Autodesk Inventor part; units mm, degrees
(part 2 of 3)
sketch "Sketch4" plane through (360.9, 0, 0) normal (0, 0, 1) x (1, 0, 0)
  line L0 (43.995, -13.335) -> (40.185, -13.335) projected
  line L1 (40.185, -13.335) -> (40.185, -1.905) projected
  line L2 (40.185, -1.905) -> (43.995, -1.905) projected
  line L3 (43.995, -1.905) -> (43.995, -13.335) projected
  circle A0 centre (38.28, -15.24) radius 1.078 projected
  circle A1 centre (45.9, 0) radius 1.078 projected
  circle A2 centre (45.9, -15.24) radius 1.078 projected
  circle A3 centre (38.28, 0) radius 1.078 projected
  line L4 (55.005, -48.5) -> (57.005, -48.5) projected
  line L5 (57.005, -48.5) -> (57.005, -45) projected
  line L6 (57.005, -45) -> (60.18, -45) projected
  line L7 (60.18, -45) -> (60.18, -35) projected
  line L8 (60.18, -35) -> (57.005, -35) projected
  line L9 (57.005, -35) -> (57.005, -25) projected
  line L10 (57.005, -25) -> (60.18, -25) projected
  line L11 (60.18, -25) -> (60.18, -15) projected
  line L12 (60.18, -15) -> (57.005, -15) projected
  line L13 (57.005, -15) -> (57.005, -5) projected
  line L14 (57.005, -5) -> (60.18, -5) projected
  line L15 (60.18, -5) -> (60.18, 5) projected
  line L16 (60.18, 5) -> (57.005, 5) projected
  line L17 (57.005, 5) -> (57.005, 15) projected
  line L18 (57.005, 15) -> (60.18, 15) projected
  line L19 (60.18, 15) -> (60.18, 25) projected
  line L20 (60.18, 25) -> (57.005, 25) projected
  line L21 (57.005, 25) -> (57.005, 35) projected
  line L22 (57.005, 35) -> (60.18, 35) projected
  line L23 (60.18, 35) -> (60.18, 45) projected
  line L24 (60.18, 45) -> (57.005, 45) projected
  line L25 (57.005, 45) -> (57.005, 48.5) projected
  line L26 (57.005, 48.5) -> (55.005, 48.5) projected
  line L27 (55.005, 48.5) -> (55.005, 47.25) projected
  line L28 (55.005, 47.25) -> (52.505, 47.25) projected
  line L29 (52.505, 47.25) -> (52.505, 48.5) projected
  line L30 (52.505, 48.5) -> (46.18, 48.5) projected
  line L31 (46.18, 48.5) -> (46.18, 51.5) projected
  line L32 (46.18, 51.5) -> (52.505, 51.5) projected
  line L33 (52.505, 51.5) -> (52.505, 52.75) projected
  line L34 (52.505, 52.75) -> (55.005, 52.75) projected
  line L35 (55.005, 52.75) -> (55.005, 51.5) projected
  line L36 (55.005, 51.5) -> (57.005, 51.5) projected
  line L37 (57.005, 51.5) -> (57.005, 55) projected
  line L38 (57.005, 55) -> (60.18, 55) projected
  line L39 (60.18, 55) -> (60.18, 65) projected
  line L40 (60.18, 65) -> (57.005, 65) projected
  line L41 (57.005, 65) -> (57.005, 75) projected
  line L42 (57.005, 75) -> (60.18, 75) projected
  line L43 (60.18, 75) -> (60.18, 86.825) projected
  line L44 (55.18, 86.825) -> (60.18, 86.825) projected
  line L45 (55.18, 90) -> (55.18, 86.825) projected
  line L46 (45.18, 90) -> (55.18, 90) projected
  line L47 (45.18, 86.825) -> (45.18, 90) projected
  line L48 (45.18, 86.825) -> (35.18, 86.825) projected
  line L49 (35.18, 90) -> (35.18, 86.825) projected
  line L50 (25.18, 90) -> (35.18, 90) projected
  line L51 (25.18, 86.825) -> (25.18, 90) projected
  line L52 (25.18, 86.825) -> (15.18, 86.825) projected
  line L53 (15.18, 90) -> (15.18, 86.825) projected
  line L54 (5.18, 90) -> (15.18, 90) projected
  line L55 (5.18, 86.825) -> (5.18, 90) projected
  line L56 (5.18, 86.825) -> (-4.82, 86.825) projected
  line L57 (-4.82, 90) -> (-4.82, 86.825) projected
  line L58 (-14.82, 90) -> (-4.82, 90) projected
  line L59 (-14.82, 86.825) -> (-14.82, 90) projected
  line L60 (-14.82, 86.825) -> (-24.82, 86.825) projected
  line L61 (-24.82, 90) -> (-24.82, 86.825) projected
  line L62 (-34.82, 90) -> (-24.82, 90) projected
  line L63 (-34.82, 86.825) -> (-34.82, 90) projected
  line L64 (-34.82, 86.825) -> (-44.82, 86.825) projected
  line L65 (-44.82, 90) -> (-44.82, 86.825) projected
  line L66 (-54.82, 90) -> (-44.82, 90) projected
  line L67 (-54.82, 86.825) -> (-54.82, 90) projected
  line L68 (-54.82, 86.825) -> (-59.82, 86.825) projected
  line L69 (-59.82, 75) -> (-59.82, 86.825) projected
  line L70 (-56.645, 75) -> (-59.82, 75) projected
  line L71 (-56.645, 75) -> (-56.645, 65) projected
  line L72 (-59.82, 65) -> (-56.645, 65) projected
  line L73 (-59.82, 55) -> (-59.82, 65) projected
  line L74 (-56.645, 55) -> (-59.82, 55) projected
  line L75 (-56.645, 55) -> (-56.645, 45) projected
  line L76 (-59.82, 45) -> (-56.645, 45) projected
  line L77 (-59.82, 35) -> (-59.82, 45) projected
  line L78 (-56.645, 35) -> (-59.82, 35) projected
  line L79 (-56.645, 35) -> (-56.645, 25) projected
  line L80 (-59.82, 25) -> (-56.645, 25) projected
  line L81 (-59.82, 15) -> (-59.82, 25) projected
  line L82 (-56.645, 15) -> (-59.82, 15) projected
  line L83 (-56.645, 15) -> (-56.645, 5) projected
  line L84 (-59.82, 5) -> (-56.645, 5) projected
  line L85 (-59.82, -5) -> (-59.82, 5) projected
  line L86 (-56.645, -5) -> (-59.82, -5) projected
  line L87 (-56.645, -5) -> (-56.645, -15) projected
  line L88 (-59.82, -15) -> (-56.645, -15) projected
  line L89 (-59.82, -25) -> (-59.82, -15) projected
  line L90 (-56.645, -25) -> (-59.82, -25) projected
  line L91 (-56.645, -25) -> (-56.645, -35) projected
  line L92 (-59.82, -35) -> (-56.645, -35) projected
  line L93 (-59.82, -45) -> (-59.82, -35) projected
  line L94 (-56.645, -45) -> (-59.82, -45) projected
  line L95 (-56.645, -45) -> (-56.645, -55) projected
  line L96 (-59.82, -55) -> (-56.645, -55) projected
  line L97 (-59.82, -65) -> (-59.82, -55) projected
  line L98 (-56.645, -65) -> (-59.82, -65) projected
  line L99 (-56.645, -65) -> (-56.645, -75) projected
  line L100 (-59.82, -75) -> (-56.645, -75) projected
  line L101 (-59.82, -75) -> (-59.82, -86.825) projected
  line L102 (-59.82, -86.825) -> (-54.82, -86.825) projected
  line L103 (-54.82, -86.825) -> (-54.82, -90) projected
  line L104 (-54.82, -90) -> (-44.82, -90) projected
  line L105 (-44.82, -90) -> (-44.82, -86.825) projected
  line L106 (-44.82, -86.825) -> (-34.82, -86.825) projected
  line L107 (-34.82, -86.825) -> (-34.82, -90) projected
  line L108 (-34.82, -90) -> (-24.82, -90) projected
  line L109 (-24.82, -90) -> (-24.82, -86.825) projected
  line L110 (-24.82, -86.825) -> (-14.82, -86.825) projected
  line L111 (-14.82, -86.825) -> (-14.82, -90) projected
  line L112 (-14.82, -90) -> (-4.82, -90) projected
  line L113 (-4.82, -90) -> (-4.82, -86.825) projected
  line L114 (-4.82, -86.825) -> (5.18, -86.825) projected
  line L115 (5.18, -86.825) -> (5.18, -90) projected
  line L116 (5.18, -90) -> (15.18, -90) projected
  line L117 (15.18, -90) -> (15.18, -86.825) projected
  line L118 (15.18, -86.825) -> (25.18, -86.825) projected
  line L119 (25.18, -86.825) -> (25.18, -90) projected
  line L120 (25.18, -90) -> (35.18, -90) projected
  line L121 (35.18, -90) -> (35.18, -86.825) projected
  line L122 (35.18, -86.825) -> (45.18, -86.825) projected
  line L123 (45.18, -86.825) -> (45.18, -90) projected
  line L124 (45.18, -90) -> (55.18, -90) projected
  line L125 (55.18, -90) -> (55.18, -86.825) projected
  line L126 (55.18, -86.825) -> (60.18, -86.825) projected
  line L127 (60.18, -86.825) -> (60.18, -75) projected
  line L128 (60.18, -75) -> (57.005, -75) projected
  line L129 (57.005, -75) -> (57.005, -65) projected
  line L130 (57.005, -65) -> (60.18, -65) projected
  line L131 (60.18, -65) -> (60.18, -55) projected
  line L132 (60.18, -55) -> (57.005, -55) projected
  line L133 (57.005, -55) -> (57.005, -51.5) projected
  line L134 (57.005, -51.5) -> (55.005, -51.5) projected
  line L135 (55.005, -51.5) -> (55.005, -52.75) projected
  line L136 (55.005, -52.75) -> (52.505, -52.75) projected
  line L137 (52.505, -52.75) -> (52.505, -51.5) projected
  line L138 (52.505, -51.5) -> (46.18, -51.5) projected
  line L139 (46.18, -51.5) -> (46.18, -48.5) projected
  line L140 (46.18, -48.5) -> (52.505, -48.5) projected
  line L141 (52.505, -48.5) -> (52.505, -47.25) projected
  line L142 (52.505, -47.25) -> (55.005, -47.25) projected
  line L143 (55.005, -47.25) -> (55.005, -48.5) projected
  circle A4 centre (23.1772, -27.4451) radius 3 projected
  circle A5 centre (-22.8172, 54) radius 3 projected
  circle A6 centre (23.1772, 27.4451) radius 3 projected
  circle A7 centre (-22.8172, -54) radius 3 projected
  circle A8 centre (-14.82, 8.175) radius 11 projected
  line L144 (45.06, 90.12) -> (55.3, 90.12)
  line L145 (55.3, 90.12) -> (55.3, 86.945)
  line L146 (55.3, 86.945) -> (60.3, 86.945)
  line L147 (60.3, 86.945) -> (60.3, 74.88)
  line L148 (60.3, 74.88) -> (57.125, 74.88)
  line L149 (57.125, 74.88) -> (57.125, 65.12)
  line L150 (57.125, 65.12) -> (60.3, 65.12)
  line L151 (60.3, 65.12) -> (60.3, 54.88)
  line L152 (60.3, 54.88) -> (57.125, 54.88)
  line L153 (57.125, 54.88) -> (57.125, 51.38)
  line L154 (57.125, 51.38) -> (54.885, 51.38)
  line L155 (54.885, 51.38) -> (54.885, 52.63)
  line L156 (54.885, 52.63) -> (52.625, 52.63)
  line L157 (52.625, 52.63) -> (52.625, 51.38)
  line L158 (52.625, 51.38) -> (46.3, 51.38)
  line L159 (46.3, 51.38) -> (46.3, 48.62)
  line L160 (46.3, 48.62) -> (52.625, 48.62)
  line L161 (52.625, 48.62) -> (52.625, 47.37)
  line L162 (52.625, 47.37) -> (54.885, 47.37)
  line L163 (54.885, 47.37) -> (54.885, 48.62)
  line L164 (54.885, 48.62) -> (57.125, 48.62)
  line L165 (57.125, 48.62) -> (57.125, 45.12)
  line L166 (57.125, 45.12) -> (60.3, 45.12)
  line L167 (60.3, 45.12) -> (60.3, 34.88)
  line L168 (60.3, 34.88) -> (57.125, 34.88)
  line L169 (57.125, 34.88) -> (57.125, 25.12)
  line L170 (57.125, 25.12) -> (60.3, 25.12)
  line L171 (60.3, 25.12) -> (60.3, 14.88)
  line L172 (60.3, 14.88) -> (57.125, 14.88)
  line L173 (57.125, 14.88) -> (57.125, 5.12)
  line L174 (57.125, 5.12) -> (60.3, 5.12)
  line L175 (60.3, 5.12) -> (60.3, -5.12)
  line L176 (60.3, -5.12) -> (57.125, -5.12)
  line L177 (57.125, -5.12) -> (57.125, -14.88)
  line L178 (57.125, -14.88) -> (60.3, -14.88)
  line L179 (60.3, -14.88) -> (60.3, -25.12)
  line L180 (60.3, -25.12) -> (57.125, -25.12)
  line L181 (57.125, -25.12) -> (57.125, -34.88)
  line L182 (57.125, -34.88) -> (60.3, -34.88)
  line L183 (60.3, -34.88) -> (60.3, -45.12)
  line L184 (60.3, -45.12) -> (57.125, -45.12)
  line L185 (57.125, -45.12) -> (57.125, -48.62)
  line L186 (57.125, -48.62) -> (54.885, -48.62)
  line L187 (54.885, -48.62) -> (54.885, -47.37)
  line L188 (54.885, -47.37) -> (52.625, -47.37)
  line L189 (52.625, -47.37) -> (52.625, -48.62)
  line L190 (52.625, -48.62) -> (46.3, -48.62)
  line L191 (46.3, -48.62) -> (46.3, -51.38)
  line L192 (46.3, -51.38) -> (52.625, -51.38)
  line L193 (52.625, -51.38) -> (52.625, -52.63)
  line L194 (52.625, -52.63) -> (54.885, -52.63)
  line L195 (54.885, -52.63) -> (54.885, -51.38)
  line L196 (54.885, -51.38) -> (57.125, -51.38)
  line L197 (57.125, -51.38) -> (57.125, -54.88)
  line L198 (57.125, -54.88) -> (60.3, -54.88)
  line L199 (60.3, -54.88) -> (60.3, -65.12)
  line L200 (60.3, -65.12) -> (57.125, -65.12)
  line L201 (57.125, -65.12) -> (57.125, -74.88)
  line L202 (57.125, -74.88) -> (60.3, -74.88)
  line L203 (60.3, -74.88) -> (60.3, -86.945)
  line L204 (60.3, -86.945) -> (55.3, -86.945)
  line L205 (55.3, -86.945) -> (55.3, -90.12)
  line L206 (55.3, -90.12) -> (45.06, -90.12)
  line L207 (45.06, -90.12) -> (45.06, -86.945)
  line L208 (45.06, -86.945) -> (35.3, -86.945)
  line L209 (35.3, -86.945) -> (35.3, -90.12)
  line L210 (35.3, -90.12) -> (25.06, -90.12)
  line L211 (25.06, -90.12) -> (25.06, -86.945)
  line L212 (25.06, -86.945) -> (15.3, -86.945)
  line L213 (15.3, -86.945) -> (15.3, -90.12)
  line L214 (15.3, -90.12) -> (5.06, -90.12)
  line L215 (5.06, -90.12) -> (5.06, -86.945)
  line L216 (5.06, -86.945) -> (-4.7, -86.945)
  line L217 (-4.7, -86.945) -> (-4.7, -90.12)
  line L218 (-4.7, -90.12) -> (-14.94, -90.12)
  line L219 (-14.94, -90.12) -> (-14.94, -86.945)
  line L220 (-14.94, -86.945) -> (-24.7, -86.945)
  line L221 (-24.7, -86.945) -> (-24.7, -90.12)
  line L222 (-24.7, -90.12) -> (-34.94, -90.12)
  line L223 (-34.94, -90.12) -> (-34.94, -86.945)
  line L224 (-34.94, -86.945) -> (-44.7, -86.945)
  line L225 (-44.7, -86.945) -> (-44.7, -90.12)
  line L226 (-44.7, -90.12) -> (-54.94, -90.12)
  line L227 (-54.94, -90.12) -> (-54.94, -86.945)
  line L228 (-54.94, -86.945) -> (-59.94, -86.945)
  line L229 (-59.94, -86.945) -> (-59.94, -74.88)
  line L230 (-59.94, -74.88) -> (-56.765, -74.88)
  line L231 (-56.765, -74.88) -> (-56.765, -65.12)
  line L232 (-56.765, -65.12) -> (-59.94, -65.12)
  line L233 (-59.94, -65.12) -> (-59.94, -54.88)
  line L234 (-59.94, -54.88) -> (-56.765, -54.88)
  line L235 (-56.765, -54.88) -> (-56.765, -45.12)
  line L236 (-56.765, -45.12) -> (-59.94, -45.12)
  line L237 (-59.94, -45.12) -> (-59.94, -34.88)
  line L238 (-59.94, -34.88) -> (-56.765, -34.88)
  line L239 (-56.765, -34.88) -> (-56.765, -25.12)
  line L240 (-56.765, -25.12) -> (-59.94, -25.12)
  line L241 (-59.94, -25.12) -> (-59.94, -14.88)
  line L242 (-59.94, -14.88) -> (-56.765, -14.88)
  line L243 (-56.765, -14.88) -> (-56.765, -5.12)
  line L244 (-56.765, -5.12) -> (-59.94, -5.12)
  line L245 (-59.94, -5.12) -> (-59.94, 5.12)
  line L246 (-59.94, 5.12) -> (-56.765, 5.12)
  line L247 (-56.765, 5.12) -> (-56.765, 14.88)
  line L248 (-56.765, 14.88) -> (-59.94, 14.88)
  line L249 (-59.94, 14.88) -> (-59.94, 25.12)
  line L250 (-59.94, 25.12) -> (-56.765, 25.12)
  line L251 (-56.765, 25.12) -> (-56.765, 34.88)
  line L252 (-56.765, 34.88) -> (-59.94, 34.88)
  line L253 (-59.94, 34.88) -> (-59.94, 45.12)
  line L254 (-59.94, 45.12) -> (-56.765, 45.12)
  line L255 (-56.765, 45.12) -> (-56.765, 54.88)
  line L256 (-56.765, 54.88) -> (-59.94, 54.88)
  line L257 (-59.94, 54.88) -> (-59.94, 65.12)
  line L258 (-59.94, 65.12) -> (-56.765, 65.12)
  line L259 (-56.765, 65.12) -> (-56.765, 74.88)
  line L260 (-56.765, 74.88) -> (-59.94, 74.88)
  line L261 (-59.94, 74.88) -> (-59.94, 86.945)
  line L262 (-59.94, 86.945) -> (-54.94, 86.945)
  line L263 (-54.94, 86.945) -> (-54.94, 90.12)
  line L264 (-54.94, 90.12) -> (-44.7, 90.12)
  line L265 (-44.7, 90.12) -> (-44.7, 86.945)
  line L266 (-44.7, 86.945) -> (-34.94, 86.945)
  line L267 (-34.94, 86.945) -> (-34.94, 90.12)
  line L268 (-34.94, 90.12) -> (-24.7, 90.12)
  line L269 (-24.7, 90.12) -> (-24.7, 86.945)
  line L270 (-24.7, 86.945) -> (-14.94, 86.945)
  line L271 (-14.94, 86.945) -> (-14.94, 90.12)
  line L272 (-14.94, 90.12) -> (-4.7, 90.12)
  line L273 (-4.7, 90.12) -> (-4.7, 86.945)
  line L274 (-4.7, 86.945) -> (5.06, 86.945)
  line L275 (5.06, 86.945) -> (5.06, 90.12)
  line L276 (5.06, 90.12) -> (15.3, 90.12)
  line L277 (15.3, 90.12) -> (15.3, 86.945)
  line L278 (15.3, 86.945) -> (25.06, 86.945)
  line L279 (25.06, 86.945) -> (25.06, 90.12)
  line L280 (25.06, 90.12) -> (35.3, 90.12)
  line L281 (35.3, 90.12) -> (35.3, 86.945)
  line L282 (35.3, 86.945) -> (45.06, 86.945)
  line L283 (45.06, 86.945) -> (45.06, 90.12)
  circle A9 centre (45.9, 0) radius 0.958
  circle A10 centre (38.28, 0) radius 1.198
  line L284 (43.875, -13.215) -> (40.305, -13.215)
  line L285 (40.305, -13.215) -> (40.305, -2.025)
  line L286 (40.305, -2.025) -> (43.875, -2.025)
  line L287 (43.875, -2.025) -> (43.875, -13.215)
  circle A11 centre (45.9, -15.24) radius 0.958
  circle A12 centre (38.28, -15.24) radius 0.958
  circle A13 centre (23.1772, -27.4451) radius 2.88
  circle A14 centre (23.1772, 27.4451) radius 2.88
  circle A15 centre (-14.82, 8.175) radius 10.88
  circle A16 centre (-22.8172, -54) radius 2.88
  circle A17 centre (-22.8172, 54) radius 2.88
  point P0 (-360.9, 0)
  dimension "d28" = 0.12
  dimension "d29" = 0.12
  dimension "d30" = 0.12
  dimension "d31" = 0.12
  dimension "d32" = 0.12
  dimension "d33" = 0.12
  dimension "d34" = 0.12
  dimension "d35" = 0.12
  dimension "d36" = 0.12
  dimension "d37" = 0.12
  dimension "d38" = 0.12
  constraints: 288 end point, 9 centre point, 142 other
  measures "d28" distance between parallel lines of L47 L283
  measures "d29" radial gap between concentric circles of A1 A9
  measures "d30" radial gap between concentric circles of A3 A10
  measures "d31" distance between parallel lines of L3 L287
  measures "d32" radial gap between concentric circles of A2 A11
  measures "d33" radial gap between concentric circles of A0 A12
  measures "d34" radial gap between concentric circles of A4 A13
  measures "d35" radial gap between concentric circles of A6 A14
  measures "d36" radial gap between concentric circles of A8 A15
  measures "d37" radial gap between concentric circles of A7 A16
  measures "d38" radial gap between concentric circles of A5 A17
extrude "Extrusion4" add sketch "Sketch4" along normal blind 3.175 contours L0 L1 L2 L3 | A0 | A1 | A2 | L143 L142 L141 L140 L139 L138 L137 L136 L135 L134 L133 L132 L131 L130 L129 L128 L127 L126 L125 L124 L123 L122 L121 L120 L119 L118 L117 L116 L115 L114 L113 L112 L111 L110 L109 L108 L107 L106 L105 L104 L103 L102 L101 L100 L99 L98 L97 L96 L95 L94 L93 L92 L91 L90 L89 L88 L87 L86 L85 L84 L83 L82 L81 L80 L79 L78 L77 L76 L75 L74 L73 L72 L71 L70 L69 L68 L67 L66 L65 L64 L63 L62 L61 L60 L59 L58 L57 L56 L55 L54 L53 L52 L51 L50 L49 L48 L47 L46 L45 L44 L43 L42 L41 L40 L39 L38 L37 L36 L35 L34 L33 L32 L31 L30 L29 L28 L27 L26 L25 L24 L23 L22 L21 L20 L19 L18 L17 L16 L15 L14 L13 L12 L11 L10 L9 L8 L7 L6 L5 L4 | A4 | A5 | A6 | A7 | A8 | A10
ref_plane "Work Plane4" through (120.3, -150.3, 0) normal (0, 0, 1) x (0, -1, 0)
sketch "Sketch5" plane through (120.3, -150.3, 0) normal (0, 0, 1) x (0, -1, 0)
  line L0 (56.885, 55.06) -> (60.06, 55.06) projected
  line L1 (60.06, 55.06) -> (60.06, 60.06) projected
  line L2 (60.06, 60.06) -> (55.06, 60.06) projected
  line L3 (55.06, 60.06) -> (55.06, 56.885) projected
  line L4 (55.06, 56.885) -> (45.06, 56.885) projected
  line L5 (45.06, 56.885) -> (45.06, 60.06) projected
  line L6 (45.06, 60.06) -> (35.06, 60.06) projected
  line L7 (35.06, 60.06) -> (35.06, 56.885) projected
  line L8 (35.06, 56.885) -> (25.06, 56.885) projected
  line L9 (25.06, 56.885) -> (25.06, 60.06) projected
  line L10 (25.06, 60.06) -> (15.06, 60.06) projected
  line L11 (15.06, 60.06) -> (15.06, 56.885) projected
  line L12 (15.06, 56.885) -> (5.06, 56.885) projected
  line L13 (5.06, 56.885) -> (5.06, 60.06) projected
  line L14 (5.06, 60.06) -> (-4.94, 60.06) projected
  line L15 (-4.94, 60.06) -> (-4.94, 56.885) projected
  line L16 (-4.94, 56.885) -> (-14.94, 56.885) projected
  line L17 (-14.94, 56.885) -> (-14.94, 60.06) projected
  line L18 (-14.94, 60.06) -> (-24.94, 60.06) projected
  line L19 (-24.94, 60.06) -> (-24.94, 56.885) projected
  line L20 (-24.94, 56.885) -> (-34.94, 56.885) projected
  line L21 (-34.94, 56.885) -> (-34.94, 60.06) projected
  line L22 (-34.94, 60.06) -> (-44.94, 60.06) projected
  line L23 (-44.94, 60.06) -> (-44.94, 56.885) projected
  line L24 (-44.94, 56.885) -> (-54.94, 56.885) projected
  line L25 (-54.94, 56.885) -> (-54.94, 60.06) projected
  line L26 (-54.94, 60.06) -> (-59.94, 60.06) projected
  line L27 (-59.94, 60.06) -> (-59.94, 55.06) projected
  line L28 (-59.94, 55.06) -> (-56.765, 55.06) projected
  line L29 (-56.765, 55.06) -> (-56.765, 45.06) projected
  line L30 (-56.765, 45.06) -> (-59.94, 45.06) projected
  line L31 (-59.94, 45.06) -> (-59.94, 35.06) projected
  line L32 (-59.94, 35.06) -> (-56.765, 35.06) projected
  line L33 (-56.765, 35.06) -> (-56.765, 25.06) projected
  line L34 (-56.765, 25.06) -> (-59.94, 25.06) projected
  line L35 (-59.94, 25.06) -> (-59.94, 15.06) projected
  line L36 (-59.94, 15.06) -> (-56.765, 15.06) projected
  line L37 (-56.765, 15.06) -> (-56.765, 5.06) projected
  line L38 (-56.765, 5.06) -> (-59.94, 5.06) projected
  line L39 (-59.94, 5.06) -> (-59.94, -4.94) projected
  line L40 (-59.94, -4.94) -> (-56.765, -4.94) projected
  line L41 (-56.765, -4.94) -> (-56.765, -14.94) projected
  line L42 (-56.765, -14.94) -> (-59.94, -14.94) projected
  line L43 (-59.94, -14.94) -> (-59.94, -24.94) projected
  line L44 (-59.94, -24.94) -> (-56.765, -24.94) projected
  line L45 (-56.765, -24.94) -> (-56.765, -34.94) projected
  line L46 (-56.765, -34.94) -> (-59.94, -34.94) projected
  line L47 (-59.94, -34.94) -> (-59.94, -44.94) projected
  line L48 (-59.94, -44.94) -> (-56.765, -44.94) projected
  line L49 (-56.765, -44.94) -> (-56.765, -54.94) projected
  line L50 (-56.765, -54.94) -> (-59.94, -54.94) projected
  line L51 (-59.94, -54.94) -> (-59.94, -59.94) projected
  line L52 (-59.94, -59.94) -> (-54.94, -59.94) projected
  line L53 (-54.94, -59.94) -> (-54.94, -56.765) projected
  line L54 (-54.94, -56.765) -> (-44.94, -56.765) projected
  line L55 (-44.94, -56.765) -> (-44.94, -59.94) projected
  line L56 (-44.94, -59.94) -> (-34.94, -59.94) projected
  line L57 (-34.94, -59.94) -> (-34.94, -56.765) projected
  line L58 (-34.94, -56.765) -> (-24.94, -56.765) projected
  line L59 (-24.94, -56.765) -> (-24.94, -59.94) projected
  line L60 (-24.94, -59.94) -> (-14.94, -59.94) projected
  line L61 (-14.94, -59.94) -> (-14.94, -56.765) projected
  line L62 (-14.94, -56.765) -> (-4.94, -56.765) projected
  line L63 (-4.94, -56.765) -> (-4.94, -59.94) projected
  line L64 (-4.94, -59.94) -> (5.06, -59.94) projected
  line L65 (5.06, -59.94) -> (5.06, -56.765) projected
  line L66 (5.06, -56.765) -> (15.06, -56.765) projected
  line L67 (15.06, -56.765) -> (15.06, -59.94) projected
  line L68 (15.06, -59.94) -> (25.06, -59.94) projected
  line L69 (25.06, -59.94) -> (25.06, -56.765) projected
  line L70 (25.06, -56.765) -> (35.06, -56.765) projected
  line L71 (35.06, -56.765) -> (35.06, -59.94) projected
  line L72 (35.06, -59.94) -> (45.06, -59.94) projected
  line L73 (45.06, -59.94) -> (45.06, -56.765) projected
  line L74 (45.06, -56.765) -> (55.06, -56.765) projected
  line L75 (55.06, -56.765) -> (55.06, -59.94) projected
  line L76 (55.06, -59.94) -> (60.06, -59.94) projected
  line L77 (60.06, -59.94) -> (60.06, -54.94) projected
  line L78 (60.06, -54.94) -> (56.885, -54.94) projected
  line L79 (56.885, -54.94) -> (56.885, -44.94) projected
  line L80 (56.885, -44.94) -> (60.06, -44.94) projected
  line L81 (60.06, -44.94) -> (60.06, -34.94) projected
  line L82 (60.06, -34.94) -> (56.885, -34.94) projected
  line L83 (56.885, -34.94) -> (56.885, -24.94) projected
  line L84 (56.885, -24.94) -> (60.06, -24.94) projected
  line L85 (60.06, -24.94) -> (60.06, -14.94) projected
  line L86 (60.06, -14.94) -> (56.885, -14.94) projected
  line L87 (56.885, -14.94) -> (56.885, -4.94) projected
  line L88 (56.885, -4.94) -> (60.06, -4.94) projected
  line L89 (60.06, -4.94) -> (60.06, 5.06) projected
  line L90 (60.06, 5.06) -> (56.885, 5.06) projected
  line L91 (56.885, 5.06) -> (56.885, 15.06) projected
  line L92 (56.885, 15.06) -> (60.06, 15.06) projected
  line L93 (60.06, 15.06) -> (60.06, 25.06) projected
  line L94 (60.06, 25.06) -> (56.885, 25.06) projected
  line L95 (56.885, 25.06) -> (56.885, 35.06) projected
  line L96 (56.885, 35.06) -> (60.06, 35.06) projected
  line L97 (60.06, 35.06) -> (60.06, 45.06) projected
  line L98 (60.06, 45.06) -> (56.885, 45.06) projected
  line L99 (56.885, 45.06) -> (56.885, 55.06) projected
  line L100 (57.005, -45.06) -> (57.005, -54.82)
  line L101 (57.005, -54.82) -> (60.18, -54.82)
  line L102 (60.18, -54.82) -> (60.18, -60.06)
  line L103 (60.18, -60.06) -> (54.94, -60.06)
  line L104 (54.94, -60.06) -> (54.94, -56.885)
  line L105 (54.94, -56.885) -> (45.18, -56.885)
  line L106 (45.18, -56.885) -> (45.18, -60.06)
  line L107 (45.18, -60.06) -> (34.94, -60.06)
  line L108 (34.94, -60.06) -> (34.94, -56.885)
  line L109 (34.94, -56.885) -> (25.18, -56.885)
  line L110 (25.18, -56.885) -> (25.18, -60.06)
  line L111 (25.18, -60.06) -> (14.94, -60.06)
  line L112 (14.94, -60.06) -> (14.94, -56.885)
  line L113 (14.94, -56.885) -> (5.18, -56.885)
  line L114 (5.18, -56.885) -> (5.18, -60.06)
  line L115 (5.18, -60.06) -> (-5.06, -60.06)
  line L116 (-5.06, -60.06) -> (-5.06, -56.885)
  line L117 (-5.06, -56.885) -> (-14.82, -56.885)
  line L118 (-14.82, -56.885) -> (-14.82, -60.06)
  line L119 (-14.82, -60.06) -> (-25.06, -60.06)
  line L120 (-25.06, -60.06) -> (-25.06, -56.885)
  line L121 (-25.06, -56.885) -> (-34.82, -56.885)
  line L122 (-34.82, -56.885) -> (-34.82, -60.06)
  line L123 (-34.82, -60.06) -> (-45.06, -60.06)
  line L124 (-45.06, -60.06) -> (-45.06, -56.885)
  line L125 (-45.06, -56.885) -> (-54.82, -56.885)
  line L126 (-54.82, -56.885) -> (-54.82, -60.06)
  line L127 (-54.82, -60.06) -> (-60.06, -60.06)
  line L128 (-60.06, -60.06) -> (-60.06, -54.82)
  line L129 (-60.06, -54.82) -> (-56.885, -54.82)
  line L130 (-56.885, -54.82) -> (-56.885, -45.06)
  line L131 (-56.885, -45.06) -> (-60.06, -45.06)
  line L132 (-60.06, -45.06) -> (-60.06, -34.82)
  line L133 (-60.06, -34.82) -> (-56.885, -34.82)
  line L134 (-56.885, -34.82) -> (-56.885, -25.06)
  line L135 (-56.885, -25.06) -> (-60.06, -25.06)
  line L136 (-60.06, -25.06) -> (-60.06, -14.82)
  line L137 (-60.06, -14.82) -> (-56.885, -14.82)
  line L138 (-56.885, -14.82) -> (-56.885, -5.06)
  line L139 (-56.885, -5.06) -> (-60.06, -5.06)
  line L140 (-60.06, -5.06) -> (-60.06, 5.18)
  line L141 (-60.06, 5.18) -> (-56.885, 5.18)
  line L142 (-56.885, 5.18) -> (-56.885, 14.94)
  line L143 (-56.885, 14.94) -> (-60.06, 14.94)
  line L144 (-60.06, 14.94) -> (-60.06, 25.18)
  line L145 (-60.06, 25.18) -> (-56.885, 25.18)
  line L146 (-56.885, 25.18) -> (-56.885, 34.94)
  line L147 (-56.885, 34.94) -> (-60.06, 34.94)
  line L148 (-60.06, 34.94) -> (-60.06, 45.18)
  line L149 (-60.06, 45.18) -> (-56.885, 45.18)
  line L150 (-56.885, 45.18) -> (-56.885, 54.94)
  line L151 (-56.885, 54.94) -> (-60.06, 54.94)
  line L152 (-60.06, 54.94) -> (-60.06, 60.18)
  line L153 (-60.06, 60.18) -> (-54.82, 60.18)
  line L154 (-54.82, 60.18) -> (-54.82, 57.005)
  line L155 (-54.82, 57.005) -> (-45.06, 57.005)
  line L156 (-45.06, 57.005) -> (-45.06, 60.18)
  line L157 (-45.06, 60.18) -> (-34.82, 60.18)
  line L158 (-34.82, 60.18) -> (-34.82, 57.005)
  line L159 (-34.82, 57.005) -> (-25.06, 57.005)
  line L160 (-25.06, 57.005) -> (-25.06, 60.18)
  line L161 (-25.06, 60.18) -> (-14.82, 60.18)
  line L162 (-14.82, 60.18) -> (-14.82, 57.005)
  line L163 (-14.82, 57.005) -> (-5.06, 57.005)
  line L164 (-5.06, 57.005) -> (-5.06, 60.18)
  line L165 (-5.06, 60.18) -> (5.18, 60.18)
  line L166 (5.18, 60.18) -> (5.18, 57.005)
  line L167 (5.18, 57.005) -> (14.94, 57.005)
  line L168 (14.94, 57.005) -> (14.94, 60.18)
  line L169 (14.94, 60.18) -> (25.18, 60.18)
  line L170 (25.18, 60.18) -> (25.18, 57.005)
  line L171 (25.18, 57.005) -> (34.94, 57.005)
  line L172 (34.94, 57.005) -> (34.94, 60.18)
  line L173 (34.94, 60.18) -> (45.18, 60.18)
  line L174 (45.18, 60.18) -> (45.18, 57.005)
  line L175 (45.18, 57.005) -> (54.94, 57.005)
  line L176 (54.94, 57.005) -> (54.94, 60.18)
  line L177 (54.94, 60.18) -> (60.18, 60.18)
  line L178 (60.18, 60.18) -> (60.18, 54.94)
  line L179 (60.18, 54.94) -> (57.005, 54.94)
  line L180 (57.005, 54.94) -> (57.005, 45.18)
  line L181 (57.005, 45.18) -> (60.18, 45.18)
  line L182 (60.18, 45.18) -> (60.18, 34.94)
  line L183 (60.18, 34.94) -> (57.005, 34.94)
  line L184 (57.005, 34.94) -> (57.005, 25.18)
  line L185 (57.005, 25.18) -> (60.18, 25.18)
  line L186 (60.18, 25.18) -> (60.18, 14.94)
  line L187 (60.18, 14.94) -> (57.005, 14.94)
  line L188 (57.005, 14.94) -> (57.005, 5.18)
  line L189 (57.005, 5.18) -> (60.18, 5.18)
  line L190 (60.18, 5.18) -> (60.18, -5.06)
  line L191 (60.18, -5.06) -> (57.005, -5.06)
  line L192 (57.005, -5.06) -> (57.005, -14.82)
  line L193 (57.005, -14.82) -> (60.18, -14.82)
  line L194 (60.18, -14.82) -> (60.18, -25.06)
  line L195 (60.18, -25.06) -> (57.005, -25.06)
  line L196 (57.005, -25.06) -> (57.005, -34.82)
  line L197 (57.005, -34.82) -> (60.18, -34.82)
  line L198 (60.18, -34.82) -> (60.18, -45.06)
  line L199 (60.18, -45.06) -> (57.005, -45.06)
  point P0 (-150.3, -120.3)
  dimension "d41" = 0.12
  constraints: 200 end point, 99 other
  measures "d41" distance between parallel lines of L79 L100
extrude "Extrusion5" add sketch "Sketch5" along normal blind 3.175 contours L99 L98 L97 L96 L95 L94 L93 L92 L91 L90 L89 L88 L87 L86 L85 L84 L83 L82 L81 L80 L79 L78 L77 L76 L75 L74 L73 L72 L71 L70 L69 L68 L67 L66 L65 L64 L63 L62 L61 L60 L59 L58 L57 L56 L55 L54 L53 L52 L51 L50 L49 L48 L47 L46 L45 L44 L43 L42 L41 L40 L39 L38 L37 L36 L35 L34 L33 L32 L31 L30 L29 L28 L27 L26 L25 L24 L23 L22 L21 L20 L19 L18 L17 L16 L15 L14 L13 L12 L11 L10 L9 L8 L7 L6 L5 L4 L3 L2 L1 L0 | L100 L101 L102 L103 L104 L105 L106 L107 L108 L109 L110 L111 L112 L113 L114 L115 L116 L117 L118 L119 L120 L121 L122 L123 L124 L125 L126 L127 L128 L129 L130 L131 L132 L133 L134 L135 L136 L137 L138 L139 L140 L141 L142 L143 L144 L145 L146 L147 L148 L149 L150 L151 L152 L153 L154 L155 L156 L157 L158 L159 L160 L161 L162 L163 L164 L165 L166 L167 L168 L169 L170 L171 L172 L173 L174 L175 L176 L177 L178 L179 L180 L181 L182 L183 L184 L185 L186 L187 L188 L189 L190 L191 L192 L193 L194 L195 L196 L197 L198 L199
ref_plane "Work Plane5" through (240.6, -150.3, 0) normal (0, 0, 1) x (0, -1, 0)
sketch "Sketch6" plane through (240.6, -150.3, 0) normal (0, 0, 1) x (0, -1, 0)
  line L0 (56.885, 55.12) -> (60.06, 55.12) projected
  line L1 (60.06, 55.12) -> (60.06, 60.12) projected
  line L2 (60.06, 60.12) -> (55.06, 60.12) projected
  line L3 (55.06, 60.12) -> (55.06, 56.945) projected
  line L4 (55.06, 56.945) -> (45.06, 56.945) projected
  line L5 (45.06, 56.945) -> (45.06, 60.12) projected
  line L6 (45.06, 60.12) -> (35.06, 60.12) projected
  line L7 (35.06, 60.12) -> (35.06, 56.945) projected
  line L8 (35.06, 56.945) -> (25.06, 56.945) projected
  line L9 (25.06, 56.945) -> (25.06, 60.12) projected
  line L10 (25.06, 60.12) -> (15.06, 60.12) projected
  line L11 (15.06, 60.12) -> (15.06, 56.945) projected
  line L12 (15.06, 56.945) -> (5.06, 56.945) projected
  line L13 (5.06, 56.945) -> (5.06, 60.12) projected
  line L14 (5.06, 60.12) -> (-4.94, 60.12) projected
  line L15 (-4.94, 60.12) -> (-4.94, 56.945) projected
  line L16 (-4.94, 56.945) -> (-14.94, 56.945) projected
  line L17 (-14.94, 56.945) -> (-14.94, 60.12) projected
  line L18 (-14.94, 60.12) -> (-24.94, 60.12) projected
  line L19 (-24.94, 60.12) -> (-24.94, 56.945) projected
  line L20 (-24.94, 56.945) -> (-34.94, 56.945) projected
  line L21 (-34.94, 56.945) -> (-34.94, 60.12) projected
  line L22 (-34.94, 60.12) -> (-44.94, 60.12) projected
  line L23 (-44.94, 60.12) -> (-44.94, 56.945) projected
  line L24 (-44.94, 56.945) -> (-54.94, 56.945) projected
  line L25 (-54.94, 56.945) -> (-54.94, 60.12) projected
  line L26 (-54.94, 60.12) -> (-59.94, 60.12) projected
  line L27 (-59.94, 60.12) -> (-59.94, 55.12) projected
  line L28 (-59.94, 55.12) -> (-56.765, 55.12) projected
  line L29 (-56.765, 55.12) -> (-56.765, 45.12) projected
  line L30 (-56.765, 45.12) -> (-59.94, 45.12) projected
  line L31 (-59.94, 45.12) -> (-59.94, 35.12) projected
  line L32 (-59.94, 35.12) -> (-56.765, 35.12) projected
  line L33 (-56.765, 35.12) -> (-56.765, 25.12) projected
  line L34 (-56.765, 25.12) -> (-59.94, 25.12) projected
  line L35 (-59.94, 25.12) -> (-59.94, 15.12) projected
  line L36 (-59.94, 15.12) -> (-56.765, 15.12) projected
  line L37 (-56.765, 15.12) -> (-56.765, 5.12) projected
  line L38 (-56.765, 5.12) -> (-59.94, 5.12) projected
  line L39 (-59.94, 5.12) -> (-59.94, -4.88) projected
  line L40 (-59.94, -4.88) -> (-56.765, -4.88) projected
  line L41 (-56.765, -4.88) -> (-56.765, -14.88) projected
  line L42 (-56.765, -14.88) -> (-59.94, -14.88) projected
  line L43 (-59.94, -14.88) -> (-59.94, -24.88) projected
  line L44 (-59.94, -24.88) -> (-56.765, -24.88) projected
  line L45 (-56.765, -24.88) -> (-56.765, -34.88) projected
  line L46 (-56.765, -34.88) -> (-59.94, -34.88) projected
  line L47 (-59.94, -34.88) -> (-59.94, -44.88) projected
  line L48 (-59.94, -44.88) -> (-56.765, -44.88) projected
  line L49 (-56.765, -44.88) -> (-56.765, -54.88) projected
  line L50 (-56.765, -54.88) -> (-59.94, -54.88) projected
  line L51 (-59.94, -54.88) -> (-59.94, -59.88) projected
  line L52 (-59.94, -59.88) -> (-54.94, -59.88) projected
  line L53 (-54.94, -59.88) -> (-54.94, -56.705) projected
  line L54 (-54.94, -56.705) -> (-44.94, -56.705) projected
  line L55 (-44.94, -56.705) -> (-44.94, -59.88) projected
  line L56 (-44.94, -59.88) -> (-34.94, -59.88) projected
  line L57 (-34.94, -59.88) -> (-34.94, -56.705) projected
  line L58 (-34.94, -56.705) -> (-24.94, -56.705) projected
  line L59 (-24.94, -56.705) -> (-24.94, -59.88) projected
  line L60 (-24.94, -59.88) -> (-14.94, -59.88) projected
  line L61 (-14.94, -59.88) -> (-14.94, -56.705) projected
  line L62 (-14.94, -56.705) -> (-4.94, -56.705) projected
  line L63 (-4.94, -56.705) -> (-4.94, -59.88) projected
  line L64 (-4.94, -59.88) -> (5.06, -59.88) projected
  line L65 (5.06, -59.88) -> (5.06, -56.705) projected
  line L66 (5.06, -56.705) -> (15.06, -56.705) projected
  line L67 (15.06, -56.705) -> (15.06, -59.88) projected
  line L68 (15.06, -59.88) -> (25.06, -59.88) projected
  line L69 (25.06, -59.88) -> (25.06, -56.705) projected
  line L70 (25.06, -56.705) -> (35.06, -56.705) projected
  line L71 (35.06, -56.705) -> (35.06, -59.88) projected
  line L72 (35.06, -59.88) -> (45.06, -59.88) projected
  line L73 (45.06, -59.88) -> (45.06, -56.705) projected
  line L74 (45.06, -56.705) -> (55.06, -56.705) projected
  line L75 (55.06, -56.705) -> (55.06, -59.88) projected
  line L76 (55.06, -59.88) -> (60.06, -59.88) projected
  line L77 (60.06, -59.88) -> (60.06, -54.88) projected
  line L78 (60.06, -54.88) -> (56.885, -54.88) projected
  line L79 (56.885, -54.88) -> (56.885, -44.88) projected
  line L80 (56.885, -44.88) -> (60.06, -44.88) projected
  line L81 (60.06, -44.88) -> (60.06, -34.88) projected
  line L82 (60.06, -34.88) -> (56.885, -34.88) projected
  line L83 (56.885, -34.88) -> (56.885, -24.88) projected
  line L84 (56.885, -24.88) -> (60.06, -24.88) projected
  line L85 (60.06, -24.88) -> (60.06, -14.88) projected
  line L86 (60.06, -14.88) -> (56.885, -14.88) projected
  line L87 (56.885, -14.88) -> (56.885, -4.88) projected
  line L88 (56.885, -4.88) -> (60.06, -4.88) projected
  line L89 (60.06, -4.88) -> (60.06, 5.12) projected
  line L90 (60.06, 5.12) -> (56.885, 5.12) projected
  line L91 (56.885, 5.12) -> (56.885, 15.12) projected
  line L92 (56.885, 15.12) -> (60.06, 15.12) projected
  line L93 (60.06, 15.12) -> (60.06, 25.12) projected
  line L94 (60.06, 25.12) -> (56.885, 25.12) projected
  line L95 (56.885, 25.12) -> (56.885, 35.12) projected
  line L96 (56.885, 35.12) -> (60.06, 35.12) projected
  line L97 (60.06, 35.12) -> (60.06, 45.12) projected
  line L98 (60.06, 45.12) -> (56.885, 45.12) projected
  line L99 (56.885, 45.12) -> (56.885, 55.12) projected
  line L100 (57.005, -54.76) -> (60.18, -54.76)
  line L101 (60.18, -54.76) -> (60.18, -60)
  line L102 (60.18, -60) -> (54.94, -60)
  line L103 (54.94, -60) -> (54.94, -56.825)
  line L104 (54.94, -56.825) -> (45.18, -56.825)
  line L105 (45.18, -56.825) -> (45.18, -60)
  line L106 (45.18, -60) -> (34.94, -60)
  line L107 (34.94, -60) -> (34.94, -56.825)
  line L108 (34.94, -56.825) -> (25.18, -56.825)
  line L109 (25.18, -56.825) -> (25.18, -60)
  line L110 (25.18, -60) -> (14.94, -60)
  line L111 (14.94, -60) -> (14.94, -56.825)
  line L112 (14.94, -56.825) -> (5.18, -56.825)
  line L113 (5.18, -56.825) -> (5.18, -60)
  line L114 (5.18, -60) -> (-5.06, -60)
  line L115 (-5.06, -60) -> (-5.06, -56.825)
  line L116 (-5.06, -56.825) -> (-14.82, -56.825)
  line L117 (-14.82, -56.825) -> (-14.82, -60)
  line L118 (-14.82, -60) -> (-25.06, -60)
  line L119 (-25.06, -60) -> (-25.06, -56.825)
  line L120 (-25.06, -56.825) -> (-34.82, -56.825)
  line L121 (-34.82, -56.825) -> (-34.82, -60)
  line L122 (-34.82, -60) -> (-45.06, -60)
  line L123 (-45.06, -60) -> (-45.06, -56.825)
  line L124 (-45.06, -56.825) -> (-54.82, -56.825)
  line L125 (-54.82, -56.825) -> (-54.82, -60)
  line L126 (-54.82, -60) -> (-60.06, -60)
  line L127 (-60.06, -60) -> (-60.06, -54.76)
  line L128 (-60.06, -54.76) -> (-56.885, -54.76)
  line L129 (-56.885, -54.76) -> (-56.885, -45)
  line L130 (-56.885, -45) -> (-60.06, -45)
  line L131 (-60.06, -45) -> (-60.06, -34.76)
  line L132 (-60.06, -34.76) -> (-56.885, -34.76)
  line L133 (-56.885, -34.76) -> (-56.885, -25)
  line L134 (-56.885, -25) -> (-60.06, -25)
  line L135 (-60.06, -25) -> (-60.06, -14.76)
  line L136 (-60.06, -14.76) -> (-56.885, -14.76)
  line L137 (-56.885, -14.76) -> (-56.885, -5)
  line L138 (-56.885, -5) -> (-60.06, -5)
  line L139 (-60.06, -5) -> (-60.06, 5.24)
  line L140 (-60.06, 5.24) -> (-56.885, 5.24)
  line L141 (-56.885, 5.24) -> (-56.885, 15)
  line L142 (-56.885, 15) -> (-60.06, 15)
  line L143 (-60.06, 15) -> (-60.06, 25.24)
  line L144 (-60.06, 25.24) -> (-56.885, 25.24)
  line L145 (-56.885, 25.24) -> (-56.885, 35)
  line L146 (-56.885, 35) -> (-60.06, 35)
  line L147 (-60.06, 35) -> (-60.06, 45.24)
  line L148 (-60.06, 45.24) -> (-56.885, 45.24)
  line L149 (-56.885, 45.24) -> (-56.885, 55)
  line L150 (-56.885, 55) -> (-60.06, 55)
  line L151 (-60.06, 55) -> (-60.06, 60.24)
  line L152 (-60.06, 60.24) -> (-54.82, 60.24)
  line L153 (-54.82, 60.24) -> (-54.82, 57.065)
  line L154 (-54.82, 57.065) -> (-45.06, 57.065)
  line L155 (-45.06, 57.065) -> (-45.06, 60.24)
  line L156 (-45.06, 60.24) -> (-34.82, 60.24)
  line L157 (-34.82, 60.24) -> (-34.82, 57.065)
  line L158 (-34.82, 57.065) -> (-25.06, 57.065)
  line L159 (-25.06, 57.065) -> (-25.06, 60.24)
  line L160 (-25.06, 60.24) -> (-14.82, 60.24)
  line L161 (-14.82, 60.24) -> (-14.82, 57.065)
  line L162 (-14.82, 57.065) -> (-5.06, 57.065)
  line L163 (-5.06, 57.065) -> (-5.06, 60.24)
  line L164 (-5.06, 60.24) -> (5.18, 60.24)
  line L165 (5.18, 60.24) -> (5.18, 57.065)
  line L166 (5.18, 57.065) -> (14.94, 57.065)
  line L167 (14.94, 57.065) -> (14.94, 60.24)
  line L168 (14.94, 60.24) -> (25.18, 60.24)
  line L169 (25.18, 60.24) -> (25.18, 57.065)
  line L170 (25.18, 57.065) -> (34.94, 57.065)
  line L171 (34.94, 57.065) -> (34.94, 60.24)
  line L172 (34.94, 60.24) -> (45.18, 60.24)
  line L173 (45.18, 60.24) -> (45.18, 57.065)
  line L174 (45.18, 57.065) -> (54.94, 57.065)
  line L175 (54.94, 57.065) -> (54.94, 60.24)
  line L176 (54.94, 60.24) -> (60.18, 60.24)
  line L177 (60.18, 60.24) -> (60.18, 55)
  line L178 (60.18, 55) -> (57.005, 55)
  line L179 (57.005, 55) -> (57.005, 45.24)
  line L180 (57.005, 45.24) -> (60.18, 45.24)
  line L181 (60.18, 45.24) -> (60.18, 35)
  line L182 (60.18, 35) -> (57.005, 35)
  line L183 (57.005, 35) -> (57.005, 25.24)
  line L184 (57.005, 25.24) -> (60.18, 25.24)
  line L185 (60.18, 25.24) -> (60.18, 15)
  line L186 (60.18, 15) -> (57.005, 15)
  line L187 (57.005, 15) -> (57.005, 5.24)
  line L188 (57.005, 5.24) -> (60.18, 5.24)
  line L189 (60.18, 5.24) -> (60.18, -5)
  line L190 (60.18, -5) -> (57.005, -5)
  line L191 (57.005, -5) -> (57.005, -14.76)
  line L192 (57.005, -14.76) -> (60.18, -14.76)
  line L193 (60.18, -14.76) -> (60.18, -25)
  line L194 (60.18, -25) -> (57.005, -25)
  line L195 (57.005, -25) -> (57.005, -34.76)
  line L196 (57.005, -34.76) -> (60.18, -34.76)
  line L197 (60.18, -34.76) -> (60.18, -45)
  line L198 (60.18, -45) -> (57.005, -45)
  line L199 (57.005, -45) -> (57.005, -54.76)
  point P0 (-150.3, -240.6)
  dimension "d44" = 0.12
  constraints: 200 end point, 99 other
  measures "d44" distance between parallel lines of L78 L100
extrude "Extrusion6" add sketch "Sketch6" along normal blind 3.175 contours L99 L98 L97 L96 L95 L94 L93 L92 L91 L90 L89 L88 L87 L86 L85 L84 L83 L82 L81 L80 L79 L78 L77 L76 L75 L74 L73 L72 L71 L70 L69 L68 L67 L66 L65 L64 L63 L62 L61 L60 L59 L58 L57 L56 L55 L54 L53 L52 L51 L50 L49 L48 L47 L46 L45 L44 L43 L42 L41 L40 L39 L38 L37 L36 L35 L34 L33 L32 L31 L30 L29 L28 L27 L26 L25 L24 L23 L22 L21 L20 L19 L18 L17 L16 L15 L14 L13 L12 L11 L10 L9 L8 L7 L6 L5 L4 L3 L2 L1 L0 | L100 L101 L102 L103 L104 L105 L106 L107 L108 L109 L110 L111 L112 L113 L114 L115 L116 L117 L118 L119 L120 L121 L122 L123 L124 L125 L126 L127 L128 L129 L130 L131 L132 L133 L134 L135 L136 L137 L138 L139 L140 L141 L142 L143 L144 L145 L146 L147 L148 L149 L150 L151 L152 L153 L154 L155 L156 L157 L158 L159 L160 L161 L162 L163 L164 L165 L166 L167 L168 L169 L170 L171 L172 L173 L174 L175 L176 L177 L178 L179 L180 L181 L182 L183 L184 L185 L186 L187 L188 L189 L190 L191 L192 L193 L194 L195 L196 L197 L198 L199
ref_plane "Work Plane6" through (0, -150.3, 0) normal (0, 0, 1) x (0, -1, 0)
sketch "Sketch7" plane through (0, -150.3, 0) normal (0, 0, 1) x (0, -1, 0)
  line L0 (56.885, 55) -> (60.06, 55) projected
  line L1 (60.06, 55) -> (60.06, 60) projected
  line L2 (60.06, 60) -> (55.06, 60) projected
  line L3 (55.06, 60) -> (55.06, 56.825) projected
  line L4 (55.06, 56.825) -> (45.06, 56.825) projected
  line L5 (45.06, 56.825) -> (45.06, 60) projected
  line L6 (45.06, 60) -> (35.06, 60) projected
  line L7 (35.06, 60) -> (35.06, 56.825) projected
  line L8 (35.06, 56.825) -> (25.06, 56.825) projected
  line L9 (25.06, 56.825) -> (25.06, 60) projected
  line L10 (25.06, 60) -> (15.06, 60) projected
  line L11 (15.06, 60) -> (15.06, 56.825) projected
  line L12 (15.06, 56.825) -> (5.06, 56.825) projected
  line L13 (5.06, 56.825) -> (5.06, 60) projected
  line L14 (5.06, 60) -> (-4.94, 60) projected
  line L15 (-4.94, 60) -> (-4.94, 56.825) projected
  line L16 (-4.94, 56.825) -> (-14.94, 56.825) projected
  line L17 (-14.94, 56.825) -> (-14.94, 60) projected
  line L18 (-14.94, 60) -> (-24.94, 60) projected
  line L19 (-24.94, 60) -> (-24.94, 56.825) projected
  line L20 (-24.94, 56.825) -> (-34.94, 56.825) projected
  line L21 (-34.94, 56.825) -> (-34.94, 60) projected
  line L22 (-34.94, 60) -> (-44.94, 60) projected
  line L23 (-44.94, 60) -> (-44.94, 56.825) projected
  line L24 (-44.94, 56.825) -> (-54.94, 56.825) projected
  line L25 (-54.94, 56.825) -> (-54.94, 60) projected
  line L26 (-54.94, 60) -> (-59.94, 60) projected
  line L27 (-59.94, 60) -> (-59.94, 55) projected
  line L28 (-59.94, 55) -> (-56.765, 55) projected
  line L29 (-56.765, 55) -> (-56.765, 45) projected
  line L30 (-56.765, 45) -> (-59.94, 45) projected
  line L31 (-59.94, 45) -> (-59.94, 35) projected
  line L32 (-59.94, 35) -> (-56.765, 35) projected
  line L33 (-56.765, 35) -> (-56.765, 25) projected
  line L34 (-56.765, 25) -> (-59.94, 25) projected
  line L35 (-59.94, 25) -> (-59.94, 15) projected
  line L36 (-59.94, 15) -> (-56.765, 15) projected
  line L37 (-56.765, 15) -> (-56.765, 5) projected
  line L38 (-56.765, 5) -> (-59.94, 5) projected
  line L39 (-59.94, 5) -> (-59.94, -5) projected
  line L40 (-59.94, -5) -> (-56.765, -5) projected
  line L41 (-56.765, -5) -> (-56.765, -15) projected
  line L42 (-56.765, -15) -> (-59.94, -15) projected
  line L43 (-59.94, -15) -> (-59.94, -25) projected
  line L44 (-59.94, -25) -> (-56.765, -25) projected
  line L45 (-56.765, -25) -> (-56.765, -35) projected
  line L46 (-56.765, -35) -> (-59.94, -35) projected
  line L47 (-59.94, -35) -> (-59.94, -45) projected
  line L48 (-59.94, -45) -> (-56.765, -45) projected
  line L49 (-56.765, -45) -> (-56.765, -55) projected
  line L50 (-56.765, -55) -> (-59.94, -55) projected
  line L51 (-59.94, -55) -> (-59.94, -60) projected
  line L52 (-59.94, -60) -> (-54.94, -60) projected
  line L53 (-54.94, -60) -> (-54.94, -56.825) projected
  line L54 (-54.94, -56.825) -> (-44.94, -56.825) projected
  line L55 (-44.94, -56.825) -> (-44.94, -60) projected
  line L56 (-44.94, -60) -> (-34.94, -60) projected
  line L57 (-34.94, -60) -> (-34.94, -56.825) projected
  line L58 (-34.94, -56.825) -> (-24.94, -56.825) projected
  line L59 (-24.94, -56.825) -> (-24.94, -60) projected
  line L60 (-24.94, -60) -> (-14.94, -60) projected
  line L61 (-14.94, -60) -> (-14.94, -56.825) projected
  line L62 (-14.94, -56.825) -> (-4.94, -56.825) projected
  line L63 (-4.94, -56.825) -> (-4.94, -60) projected
  line L64 (-4.94, -60) -> (5.06, -60) projected
  line L65 (5.06, -60) -> (5.06, -56.825) projected
  line L66 (5.06, -56.825) -> (15.06, -56.825) projected
  line L67 (15.06, -56.825) -> (15.06, -60) projected
  line L68 (15.06, -60) -> (25.06, -60) projected
  line L69 (25.06, -60) -> (25.06, -56.825) projected
  line L70 (25.06, -56.825) -> (35.06, -56.825) projected
  line L71 (35.06, -56.825) -> (35.06, -60) projected
  line L72 (35.06, -60) -> (45.06, -60) projected
  line L73 (45.06, -60) -> (45.06, -56.825) projected
  line L74 (45.06, -56.825) -> (55.06, -56.825) projected
  line L75 (55.06, -56.825) -> (55.06, -60) projected
  line L76 (55.06, -60) -> (60.06, -60) projected
  line L77 (60.06, -60) -> (60.06, -55) projected
  line L78 (60.06, -55) -> (56.885, -55) projected
  line L79 (56.885, -55) -> (56.885, -45) projected
  line L80 (56.885, -45) -> (60.06, -45) projected
  line L81 (60.06, -45) -> (60.06, -35) projected
  line L82 (60.06, -35) -> (56.885, -35) projected
  line L83 (56.885, -35) -> (56.885, -25) projected
  line L84 (56.885, -25) -> (60.06, -25) projected
  line L85 (60.06, -25) -> (60.06, -15) projected
  line L86 (60.06, -15) -> (56.885, -15) projected
  line L87 (56.885, -15) -> (56.885, -5) projected
  line L88 (56.885, -5) -> (60.06, -5) projected
  line L89 (60.06, -5) -> (60.06, 5) projected
  line L90 (60.06, 5) -> (56.885, 5) projected
  line L91 (56.885, 5) -> (56.885, 15) projected
  line L92 (56.885, 15) -> (60.06, 15) projected
  line L93 (60.06, 15) -> (60.06, 25) projected
  line L94 (60.06, 25) -> (56.885, 25) projected
  line L95 (56.885, 25) -> (56.885, 35) projected
  line L96 (56.885, 35) -> (60.06, 35) projected
  line L97 (60.06, 35) -> (60.06, 45) projected
  line L98 (60.06, 45) -> (56.885, 45) projected
  line L99 (56.885, 45) -> (56.885, 55) projected
  line L100 (60.18, 54.88) -> (57.005, 54.88)
  line L101 (57.005, 54.88) -> (57.005, 45.12)
  line L102 (57.005, 45.12) -> (60.18, 45.12)
  line L103 (60.18, 45.12) -> (60.18, 34.88)
  line L104 (60.18, 34.88) -> (57.005, 34.88)
  line L105 (57.005, 34.88) -> (57.005, 25.12)
  line L106 (57.005, 25.12) -> (60.18, 25.12)
  line L107 (60.18, 25.12) -> (60.18, 14.88)
  line L108 (60.18, 14.88) -> (57.005, 14.88)
  line L109 (57.005, 14.88) -> (57.005, 5.12)
  line L110 (57.005, 5.12) -> (60.18, 5.12)
  line L111 (60.18, 5.12) -> (60.18, -5.12)
  line L112 (60.18, -5.12) -> (57.005, -5.12)
  line L113 (57.005, -5.12) -> (57.005, -14.88)
  line L114 (57.005, -14.88) -> (60.18, -14.88)
  line L115 (60.18, -14.88) -> (60.18, -25.12)
  line L116 (60.18, -25.12) -> (57.005, -25.12)
  line L117 (57.005, -25.12) -> (57.005, -34.88)
  line L118 (57.005, -34.88) -> (60.18, -34.88)
  line L119 (60.18, -34.88) -> (60.18, -45.12)
  line L120 (60.18, -45.12) -> (57.005, -45.12)
  line L121 (57.005, -45.12) -> (57.005, -54.88)
  line L122 (57.005, -54.88) -> (60.18, -54.88)
  line L123 (60.18, -54.88) -> (60.18, -60.12)
  line L124 (60.18, -60.12) -> (54.94, -60.12)
  line L125 (54.94, -60.12) -> (54.94, -56.945)
  line L126 (54.94, -56.945) -> (45.18, -56.945)
  line L127 (45.18, -56.945) -> (45.18, -60.12)
  line L128 (45.18, -60.12) -> (34.94, -60.12)
  line L129 (34.94, -60.12) -> (34.94, -56.945)
  line L130 (34.94, -56.945) -> (25.18, -56.945)
  line L131 (25.18, -56.945) -> (25.18, -60.12)
  line L132 (25.18, -60.12) -> (14.94, -60.12)
  line L133 (14.94, -60.12) -> (14.94, -56.945)
  line L134 (14.94, -56.945) -> (5.18, -56.945)
  line L135 (5.18, -56.945) -> (5.18, -60.12)
  line L136 (5.18, -60.12) -> (-5.06, -60.12)
  line L137 (-5.06, -60.12) -> (-5.06, -56.945)
  line L138 (-5.06, -56.945) -> (-14.82, -56.945)
  line L139 (-14.82, -56.945) -> (-14.82, -60.12)
  line L140 (-14.82, -60.12) -> (-25.06, -60.12)
  line L141 (-25.06, -60.12) -> (-25.06, -56.945)
  line L142 (-25.06, -56.945) -> (-34.82, -56.945)
  line L143 (-34.82, -56.945) -> (-34.82, -60.12)
  line L144 (-34.82, -60.12) -> (-45.06, -60.12)
  line L145 (-45.06, -60.12) -> (-45.06, -56.945)
  line L146 (-45.06, -56.945) -> (-54.82, -56.945)
  line L147 (-54.82, -56.945) -> (-54.82, -60.12)
  line L148 (-54.82, -60.12) -> (-60.06, -60.12)
  line L149 (-60.06, -60.12) -> (-60.06, -54.88)
  line L150 (-60.06, -54.88) -> (-56.885, -54.88)
  line L151 (-56.885, -54.88) -> (-56.885, -45.12)
  line L152 (-56.885, -45.12) -> (-60.06, -45.12)
  line L153 (-60.06, -45.12) -> (-60.06, -34.88)
  line L154 (-60.06, -34.88) -> (-56.885, -34.88)
  line L155 (-56.885, -34.88) -> (-56.885, -25.12)
  line L156 (-56.885, -25.12) -> (-60.06, -25.12)
  line L157 (-60.06, -25.12) -> (-60.06, -14.88)
  line L158 (-60.06, -14.88) -> (-56.885, -14.88)
  line L159 (-56.885, -14.88) -> (-56.885, -5.12)
  line L160 (-56.885, -5.12) -> (-60.06, -5.12)
  line L161 (-60.06, -5.12) -> (-60.06, 5.12)
  line L162 (-60.06, 5.12) -> (-56.885, 5.12)
  line L163 (-56.885, 5.12) -> (-56.885, 14.88)
  line L164 (-56.885, 14.88) -> (-60.06, 14.88)
  line L165 (-60.06, 14.88) -> (-60.06, 25.12)
  line L166 (-60.06, 25.12) -> (-56.885, 25.12)
  line L167 (-56.885, 25.12) -> (-56.885, 34.88)
  line L168 (-56.885, 34.88) -> (-60.06, 34.88)
  line L169 (-60.06, 34.88) -> (-60.06, 45.12)
  line L170 (-60.06, 45.12) -> (-56.885, 45.12)
  line L171 (-56.885, 45.12) -> (-56.885, 54.88)
  line L172 (-56.885, 54.88) -> (-60.06, 54.88)
  line L173 (-60.06, 54.88) -> (-60.06, 60.12)
  line L174 (-60.06, 60.12) -> (-54.82, 60.12)
  line L175 (-54.82, 60.12) -> (-54.82, 56.945)
  line L176 (-54.82, 56.945) -> (-45.06, 56.945)
  line L177 (-45.06, 56.945) -> (-45.06, 60.12)
  line L178 (-45.06, 60.12) -> (-34.82, 60.12)
  line L179 (-34.82, 60.12) -> (-34.82, 56.945)
  line L180 (-34.82, 56.945) -> (-25.06, 56.945)
  line L181 (-25.06, 56.945) -> (-25.06, 60.12)
  line L182 (-25.06, 60.12) -> (-14.82, 60.12)
  line L183 (-14.82, 60.12) -> (-14.82, 56.945)
  line L184 (-14.82, 56.945) -> (-5.06, 56.945)
  line L185 (-5.06, 56.945) -> (-5.06, 60.12)
  line L186 (-5.06, 60.12) -> (5.18, 60.12)
  line L187 (5.18, 60.12) -> (5.18, 56.945)
  line L188 (5.18, 56.945) -> (14.94, 56.945)
  line L189 (14.94, 56.945) -> (14.94, 60.12)
  line L190 (14.94, 60.12) -> (25.18, 60.12)
  line L191 (25.18, 60.12) -> (25.18, 56.945)
  line L192 (25.18, 56.945) -> (34.94, 56.945)
  line L193 (34.94, 56.945) -> (34.94, 60.12)
  line L194 (34.94, 60.12) -> (45.18, 60.12)
  line L195 (45.18, 60.12) -> (45.18, 56.945)
  line L196 (45.18, 56.945) -> (54.94, 56.945)
  line L197 (54.94, 56.945) -> (54.94, 60.12)
  line L198 (54.94, 60.12) -> (60.18, 60.12)
  line L199 (60.18, 60.12) -> (60.18, 54.88)
  point P0 (-150.3, 0)
  dimension "d47" = 0.12
  constraints: 200 end point, 99 other
  measures "d47" distance between parallel lines of L0 L100
extrude "Extrusion7" add sketch "Sketch7" along normal blind 3.175 contours L99 L98 L97 L96 L95 L94 L93 L92 L91 L90 L89 L88 L87 L86 L85 L84 L83 L82 L81 L80 L79 L78 L77 L76 L75 L74 L73 L72 L71 L70 L69 L68 L67 L66 L65 L64 L63 L62 L61 L60 L59 L58 L57 L56 L55 L54 L53 L52 L51 L50 L49 L48 L47 L46 L45 L44 L43 L42 L41 L40 L39 L38 L37 L36 L35 L34 L33 L32 L31 L30 L29 L28 L27 L26 L25 L24 L23 L22 L21 L20 L19 L18 L17 L16 L15 L14 L13 L12 L11 L10 L9 L8 L7 L6 L5 L4 L3 L2 L1 L0 | L100 L101 L102 L103 L104 L105 L106 L107 L108 L109 L110 L111 L112 L113 L114 L115 L116 L117 L118 L119 L120 L121 L122 L123 L124 L125 L126 L127 L128 L129 L130 L131 L132 L133 L134 L135 L136 L137 L138 L139 L140 L141 L142 L143 L144 L145 L146 L147 L148 L149 L150 L151 L152 L153 L154 L155 L156 L157 L158 L159 L160 L161 L162 L163 L164 L165 L166 L167 L168 L169 L170 L171 L172 L173 L174 L175 L176 L177 L178 L179 L180 L181 L182 L183 L184 L185 L186 L187 L188 L189 L190 L191 L192 L193 L194 L195 L196 L197 L198 L199
ref_plane "Work Plane7" through (390.9, -150.3, 0) normal (0, 0, 1) x (0, 1, 0)